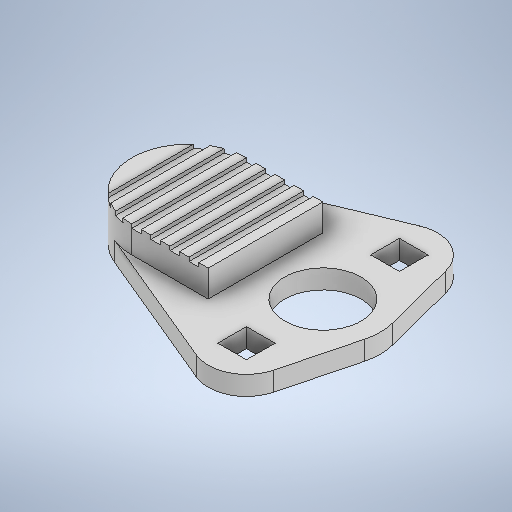
# Autodesk Inventor part: Top Frame
Saved by Autodesk Inventor 2026.2 (Build 302298010, 298A)
## iProperties
Created: 2026-05-06
Part Number: Top Frame
Material: Generic
Document SubType Name: Modeling
Designer: piete
Density: 1 g/cm^3
Appearance: Default
Author: piete
Autodesk Inventor part; units mm, degrees
ref_plane "YZ Plane" through (0, 0, 0) normal (1, 0, 0) x (0, 1, 0)
ref_plane "XZ Plane" through (0, 0, 0) normal (0, 1, 0) x (-1, 0, 0)
ref_plane "XY Plane" through (0, 0, 0) normal (0, 0, 1) x (1, 0, 0)
sketch "Sketch1" plane through (0, 0, 0) normal (0, 1, 0) x (-1, 0, 0)
  circle A0 centre (-30, 0) radius 20
  circle A1 centre (40, 0) radius 30
  circle A2 centre (-30, 0) radius 30
  circle A3 centre (-30, -40) radius 20
  circle A4 centre (-30, 40) radius 20
  line L0 (51.5385, 27.6923) -> (-22.3077, 58.4615)
  line L1 (-49.3649, 45) -> (-59.0474, 7.5)
  line L2 (-22.3077, -58.4615) -> (51.5385, -27.6923)
  line L3 (-22.5, 32.5) -> (-37.5, 32.5)
  line L4 (-37.5, 32.5) -> (-37.5, 47.5)
  line L5 (-37.5, 47.5) -> (-22.5, 47.5)
  line L6 (-22.5, 47.5) -> (-22.5, 32.5)
  line L7 (-22.5, -47.5) -> (-37.5, -47.5)
  line L8 (-37.5, -47.5) -> (-37.5, -32.5)
  line L9 (-37.5, -32.5) -> (-22.5, -32.5)
  line L10 (-22.5, -32.5) -> (-22.5, -47.5)
  line L11 (-49.3649, -45) -> (-59.0474, -7.5)
  point P0 (0, 0)
  point P1 (-57.6923, -11.5385)
  point P2 (-38.2402, -58.2236)
  point P3 (-15.4763, 26.25)
  point P4 (-15.4763, -26.25)
  point P5 (-44.5237, 26.25)
  point P6 (-44.5237, -26.25)
  point P7 (-30, 20)
  point P8 (-30, -20)
  dimension "d0" = 40
  dimension "d7" = 30
  dimension "d9" = 60
  dimension "d10" = 40
  dimension "d12" = 60
  dimension "d13" = 40
  dimension "d14" = 40
  dimension "d54" = 15
  dimension "d55" = 15
  dimension "d56" = 15
  dimension "d57" = 15
  dimension "d58" = 40
  dimension "d59" = 30
  dimension "d60" = 7.5
  dimension "d61" = 7.5
  dimension "d62" = 40
  dimension "d63" = 40
  dimension "d64" = 30
  dimension "d65" = 7.5
  dimension "d66" = 7.5
  dimension "d67" = 40
  constraints: 24 end point, 10 point on circle, 8 tangent, 5 centre point, 4 parallel, 2 horizontal, 2 perpendicular, 1 coincident
  measures "d0" diameter of A0
  measures "d7" distance of A0.centre point (0, 0)
  measures "d9" diameter of A1
  measures "d10" distance of point (0, 0) A1.centre
  measures "d12" diameter of A2
  measures "d13" diameter of A3
  measures "d14" diameter of A4
  measures "d54" distance of L4.end L5.end
  measures "d55" distance of L3.end L4.end
  measures "d56" distance of L8.end L9.end
  measures "d57" distance of L7.end L8.end
  measures "d58" vertical distance of point (0, 0) A3.centre
  measures "d59" horizontal distance of point (0, 0) A3.centre
  measures "d60" distance from line of A3.centre L7
  measures "d61" distance from line of A3.centre L8
  measures "d62" vertical distance of A3.centre A1.centre
  measures "d63" vertical distance of A1.centre A4.centre
  measures "d64" horizontal distance of A4.centre point (0, 0)
  measures "d65" distance from line of A4.centre L4
  measures "d66" distance from line of A4.centre L5
  measures "d67" distance of A4.centre A0.centre
extrude "Extrusion1" add sketch "Sketch1" along normal blind 10 contours A0 A4 A2 A3 | A0 A3 A2 A4 | A4 A2 | A3 A2 | A4 A2 | A2 L1 A4 | A4 L0 A1 L2 A3 A2 | A3 A2 | A3 L11 A2 | A1
sketch "Sketch5" plane through (0, 10, 0) normal (0, 1, 0) x (1, 0, 0)
  arc A0 (-51.5385, 27.6923) -> (-51.5385, -27.6923) centre (-40, 0) ccw projected
  circle A1 centre (-40, 0) radius 30
  line L0 (-40, 30) -> (0, 30)
  line L1 (0, 30) -> (0, -30)
  line L2 (0, -30) -> (-40, -30)
  line L3 (-40, -30) -> (-40, 30)
  point P0 (0, 0)
  point P1 (0, 0)
  dimension "d70" = 60
  dimension "d68" = 40
  dimension "d69" = 30
  dimension "d71" = 60
  constraints: 8 end point, 2 midpoint, 2 parallel, 1 coincident, 1 horizontal, 1 perpendicular, 3 other
  measures "d68" distance of point (-40, 0) point (0, 0)
  measures "d69" distance from line of point (0, 0) L0
  measures "d71" distance of L0.end L1.end
extrude "Extrusion5" add sketch "Sketch5" along normal blind 14
sketch "Sketch6" plane through (-40, 10, 30) normal (0, 0, 1) x (1, 0, 0)
  line L0 (40, 14) -> (0, 14) projected
  line L1 (40, 14) -> (35, 14)
  line L2 (35, 14) -> (35, 12)
  line L3 (35, 12) -> (40, 12)
  line L4 (40, 12) -> (40, 14)
  line L5 (30, 14) -> (25, 14)
  line L6 (25, 14) -> (25, 12)
  line L7 (25, 12) -> (30, 12)
  line L8 (30, 12) -> (30, 14)
  line L9 (20, 14) -> (15, 14)
  line L10 (15, 14) -> (15, 12)
  line L11 (15, 12) -> (20, 12)
  line L12 (20, 12) -> (20, 14)
  line L13 (10, 14) -> (5, 14)
  line L14 (5, 14) -> (5, 12)
  line L15 (5, 12) -> (10, 12)
  line L16 (10, 12) -> (10, 14)
  line L17 (0, 14) -> (-5, 14)
  line L18 (-5, 14) -> (-5, 12)
  line L19 (-5, 12) -> (0, 12)
  line L20 (0, 12) -> (0, 14)
  line L21 (-10, 14) -> (-15, 14)
  line L22 (-15, 14) -> (-15, 12)
  line L23 (-15, 12) -> (-10, 12)
  line L24 (-10, 12) -> (-10, 14)
  line L25 (-20, 14) -> (-25, 14)
  line L26 (-25, 14) -> (-25, 12)
  line L27 (-25, 12) -> (-20, 12)
  line L28 (-20, 12) -> (-20, 14)
  line L29 (-30, -10) -> (-30, 14) projected
  line L30 (-30, 14) -> (-30, 12)
  line L31 (-30, 12) -> (40, 12)
  line L32 (40, 0) -> (40, 14) projected
  line L33 (40, 14) -> (-30, 14)
  point P0 (40, -10)
  point P1 (-5, 13)
  point P2 (30, 12)
  point P3 (35, 12)
  point P4 (20, 12)
  point P5 (25, 12)
  point P6 (10, 12)
  point P7 (15, 14)
  point P8 (0, 12)
  point P9 (5, 12)
  point P10 (5, 14)
  point P11 (-5, 14)
  point P12 (-10, 12)
  point P13 (-5, 12)
  point P14 (-15, 14)
  point P15 (-20, 14)
  dimension "d74" = 5
  dimension "d75" = 2
  dimension "d76" = 5
  dimension "d77" = 2
  dimension "d78" = 5
  dimension "d79" = 2
  dimension "d80" = 5
  dimension "d81" = 2
  dimension "d82" = 5
  dimension "d83" = 2
  dimension "d84" = 5
  dimension "d85" = 2
  dimension "d86" = 5
  dimension "d87" = 2
  dimension "d88" = 5
  dimension "d89" = 5
  dimension "d90" = 5
  dimension "d91" = 5
  dimension "d92" = 5
  dimension "d93" = 5
  dimension "d94" = 2
  constraints: 62 end point, 14 parallel, 8 point on line, 7 horizontal, 7 perpendicular, 1 collinear, 1 midpoint
  measures "d74" distance of L3.end L2.end
  measures "d75" distance of L2.end L1.end
  measures "d76" distance of L7.end L6.end
  measures "d77" distance of L6.end L5.end
  measures "d78" distance of L11.end L10.end
  measures "d79" distance of L10.end L9.end
  measures "d80" distance of L15.end L14.end
  measures "d81" distance of L14.end L13.end
  measures "d82" distance of L19.end L18.end
  measures "d83" distance of L18.end L17.end
  measures "d84" distance of L23.end L22.end
  measures "d85" distance of L22.end L21.end
  measures "d86" distance of L27.end L26.end
  measures "d87" distance of L26.end L25.end
  measures "d88" distance between parallel lines of L8 L2
  measures "d89" distance between parallel lines of L6 L12
  measures "d90" distance between parallel lines of L10 L16
  measures "d91" distance between parallel lines of L14 L20
  measures "d92" distance from line of point (-5, 13) L24
  measures "d93" distance between parallel lines of L22 L28
  measures "d94" distance of L30.start L30.end
extrude "Extrusion6" cut sketch "Sketch6" against normal through all contours L2 L31 L8 L0 | L6 L31 L12 L0 | L10 L31 L16 L0 | L14 L31 L20 L0 | L18 L31 L24 L33 | L22 L31 L28 L33
equation "\"d60\" = 0.5 * d57"
equation "\"d61\" = 0.5 * d56"
equation "\"d65\" = 0.5 * d54"
equation "\"d66\" = 0.5 * d55"
body "Solid1"
